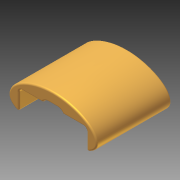
# Autodesk Inventor part: Channel - Bumper
Saved by Autodesk Inventor 2011 (Build 150239000, 239)
## iProperties
Shininess: 64.0
Length Units: 11272
Angle Units: 11279
Time Units: 11290
Mass Units: 11286
Length Display Precision: 3
Angle Display Precision: 2
Compacted: True
Part Number: Channel - Bumper
Document SubType Name: Modeling
Created: 2002-10-17
Designer: Autodesk, Inc.
Project: Inventor Samples
Density: 0.93 g/cm^3
Material: Rubber
Mass: 0.972905 g
Surface Area: 11.0236 cm^2
Volume: 1.04613 cm^3
Density: 0.0
Volumn: 0.0
Area: 0.0
PropertySet Name: Model Information
Control State: 0
Master: False
Checked Out: False
Author: Autodesk, Inc.
Revision Number: A
Autodesk Inventor part; units mm, degrees
ref_plane "YZ Plane" through (0, 0, 0) normal (1, 0, 0) x (0, 1, 0)
ref_plane "XZ Plane" through (0, 0, 0) normal (0, 1, 0) x (-1, 0, 0)
sketch "Sketch1" plane through (0, 0, 0) normal (0, 0, 1) x (1, 0, 0)
  line L0 (0, 5.406) -> (0, -9.006) projected
  line L1 (-19.4667, 0) -> (19.4667, 0) projected
  line L2 (-7.9375, -4.7752) -> (-7.9375, 0)
  line L3 (7.9375, 0) -> (7.9375, -4.7752)
  spline S0 degree 4 poles (-7.9375, -4.7752) (-8.7114, -4.4935) (-10.3313, -3.5286) (-10.6593, -1.5949) (-8.9612, 1.4328) (0.0021, 4.6919) (8.9555, 1.4468) (10.6649, -1.6102) (10.3271, -3.5171) (8.7114, -4.4935) (7.9375, -4.7752) knots 0 0 0 0 0 0.100078 0.225078 0.409682 0.590318 0.774922 0.899922 1 1 1 1 1
  line L4 (-1.9702, -6.9471) -> (-13.9048, -2.6033) construction
  arc A0 (-11.0274, -2.1186) -> (-3.8629, -4.7263) centre (-5.965, 0.6442) ccw construction
  line L5 (13.9048, -2.6033) -> (1.9702, -6.9471) construction
  arc A1 (3.912, -4.6926) -> (10.9681, -2.1244) centre (6.0313, 0.462) ccw construction
  point P0 (-10.3124, -2.4242)
  point P1 (-9.3168, 0)
  point P2 (9.3168, 0)
  point P3 (10.3124, -2.4242)
  point P4 (-7.9375, -2.3876)
  point P5 (0, 3.258)
  dimension "d1" = 4.7752
  dimension "d4" = 15.875
  dimension "d5" = 20.6248
  dimension "d6" = 70
  dimension "d7" = 70
  constraints: 8 end point, 6 point on circle, 4 midpoint, 4 point on line, 2 centre point, 2 equal length, 2 symmetric about line, 2 tangent, 1 parallel, 12 other
  measures "d1" distance of L2.start L2.end
  measures "d4" distance between parallel lines of L3 L2
  measures "d5" distance of point (10.312, -2.424) point (-10.312, -2.424)
  measures "d6" angle of L0 L4
  measures "d7" angle of L0 L5
extrude "Extrusion1" add sketch "Sketch1" along normal blind 17.4752
fillet "Fillet1" radius 0.762 2 edges at (-7.9375, 0, 8.7376) (7.9375, 0, 8.7376)
sketch "Sketch2" plane through (-7.1755, 0, 0) normal (0, -1, 0) x (1, 0, 0)
  line L0 (14.351, 17.4752) -> (0, 17.4752) projected
  line L1 (7.1755, 20.9702) -> (7.1755, -3.495) projected
  line L2 (4.7879, 17.4752) -> (9.5631, 17.4752)
  line L3 (9.5631, 17.4752) -> (9.5631, 13.5128)
  line L4 (9.5631, 13.5128) -> (4.7879, 13.5128)
  line L5 (4.7879, 13.5128) -> (4.7879, 17.4752)
  dimension "d9" = 3.9624
  dimension "d10" = 4.7752
  constraints: 8 end point, 2 parallel, 1 horizontal, 1 perpendicular, 1 point on line, 1 other
  measures "d9" distance of L4.end L2.start
  measures "d10" distance of L3.end L4.end
extrude "Extrusion2" cut sketch "Sketch2" against normal blind 0.762
fillet "Fillet2" radius 1.524 2 edges at (-2.3876, 0.762, 15.494) (2.3876, 0.762, 15.494)
fillet "Fillet3" radius 0.381 2 edges at (-7.9375, -4.7752, 8.7376) (7.9375, -4.7752, 8.7376)
fillet "Fillet5" radius 0.381 2 edges at (-2.3876, 0, 15.494) (2.3876, 0, 15.494)
fillet "Fillet4" radius 0.381 9 edges at (9.3618, -0.0494, 0) (-9.3621, -0.0497, 0) (-8.1161, -4.5239, 0) (-7.9375, -2.4816, 0) (-7.7143, -0.2232, 0) (0, 0, 0) (7.7143, -0.2232, 0) (7.9375, -2.4811, 0) (8.1165, -4.5233, 0)
fillet "Fillet4" radius 0.381 23 edges at (-9.3621, -0.0497, 17.4752) (9.3618, -0.0494, 17.4752) (8.1165, -4.5233, 17.4752) (7.9375, -2.4811, 17.4752) (7.7143, -0.2232, 17.4752) (4.8836, 0, 17.4752) (-4.8836, 0, 17.4752) (2.5005, 0.0111, 17.4752) (-2.5005, 0.0111, 17.4752) (-2.4009, 0.0513, 17.4752) (2.4009, 0.0513, 17.4752) (-2.3331, 0.1013, 17.4752) (2.3331, 0.1013, 17.4752) (-2.3876, 0.4107, 17.4752) (2.3876, 0.4107, 17.4752) (-1.7493, 0.6011, 17.4752) (1.7493, 0.6011, 17.4752) (0, 0.762, 17.4752) (-1.7277, 0.762, 17.4752) (1.7277, 0.762, 17.4752) (-7.7143, -0.2232, 17.4752) (-7.9375, -2.4816, 17.4752) (-8.1161, -4.5239, 17.4752)
ref_plane "Work Plane1" through (0, 0, 6.35) normal (0, 0, 1) x (1, 0, 0)
sketch "Sketch3" plane through (0, 0, 6.35) normal (0, 0, 1) x (1, 0, 0)
  line L0 (-7.9375, -4.2011) -> (-7.9375, -0.762) projected
  line L1 (-7.9375, -3.8201) -> (-7.1755, -2.2961)
  line L2 (-7.1755, -2.2961) -> (-7.9375, -2.2961)
  line L3 (-7.9375, -3.8201) -> (-7.9375, -2.2961)
  line L4 (-7.9375, -4.2011) -> (-8.3185, -4.2011) projected
  dimension "d19" = 1.524
  dimension "d20" = 0.762
  dimension "d21" = 0.381
  constraints: 6 end point, 2 perpendicular, 2 point on line
  measures "d19" distance of L1.start L2.end
  measures "d20" distance of L1.end L2.end
  measures "d21" distance from line of L1.start L4
extrude "Extrusion3" add sketch "Sketch3" along normal blind 3.175
mirror "Mirror1" about plane through (0, 0, 0) normal (1, 0, 0) of "Extrusion3"
equation "\"d7\" = d6"
body "Solid1"
